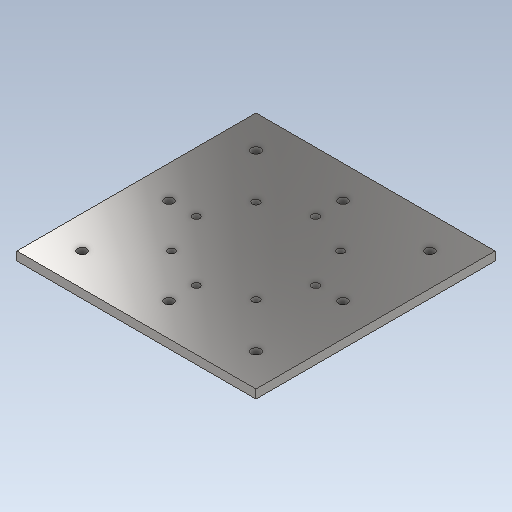
# Autodesk Inventor part: Lift.02.00.00.06
Saved by Autodesk Inventor 2021 (Build 250183000, 183)
## iProperties
Created: 2020-09-20
Part Number: Lift.02.00.00.06
Material: Сталь нержавеющая, 440C
Document SubType Name: ЛистМат
Designer: Kostya
Density: 7.75 g/cm^3
Sheet Metal Rule: По умолчанию_мм
Appearance: С умеренной полировкой
Author: Kostya
Autodesk Inventor part; units mm, degrees
ref_plane "YZ Plane" through (0, 0, 0) normal (1, 0, 0) x (0, 1, 0)
ref_plane "XZ Plane" through (0, 0, 0) normal (0, 1, 0) x (-1, 0, 0)
ref_plane "XY Plane" through (0, 0, 0) normal (0, 0, 1) x (1, 0, 0)
sketch "Эскиз1" plane through (0, 0, 0) normal (0, 1, 0) x (-1, 0, 0)
  line L0 (-275, 275) -> (275, 275)
  line L1 (275, 275) -> (275, -275)
  line L2 (275, -275) -> (-275, -275)
  line L3 (-275, -275) -> (-275, 275)
  line L4 (-275, 275) -> (275, -275) construction
  line L5 (275, 275) -> (-275, -275) construction
  circle A0 centre (200, -200) radius 10.5
  circle A1 centre (200, 0) radius 10.5
  circle A2 centre (200, 200) radius 10.5
  circle A3 centre (0, 200) radius 10.5
  circle A4 centre (-200, 200) radius 10.5
  circle A5 centre (-200, 0) radius 10.5
  circle A6 centre (-200, -200) radius 10.5
  circle A7 centre (0, -200) radius 10.5
  circle A8 centre (0, 0) radius 137.5 construction
  circle A9 centre (0, -137.5) radius 8.5
  circle A10 centre (97.2272, -97.2272) radius 8.5
  circle A11 centre (137.5, 0) radius 8.5
  circle A12 centre (97.2272, 97.2272) radius 8.5
  circle A13 centre (0, 137.5) radius 8.5
  circle A14 centre (-97.2272, 97.2272) radius 8.5
  circle A15 centre (-137.5, 0) radius 8.5
  circle A16 centre (-97.2272, -97.2272) radius 8.5
  dimension "d7" = 275
  dimension "d0" = 550
  dimension "d1" = 550
  dimension "d2" = 75
  dimension "d3" = 75
  dimension "d4" = 75
  dimension "d5" = 75
  dimension "d6" = 21
  dimension "d8" = 17
  dimension "d11" = 360
  measures "d0" distance of L1.end L2.end
  measures "d1" distance of L0.end L1.end
  measures "d2" distance from line of L2 A6.centre
  measures "d3" distance from line of L3 A6.centre
  measures "d4" distance from line of L1 A0.centre
  measures "d5" distance from line of L0 A2.centre
  measures "d6" diameter of A5
  measures "d8" diameter of A9
extrude "Пластина1" add sketch "Эскиз1" along normal blind 20
equation "\"d13\" = Толщина"
equation "\"Толщина\" = 20"
